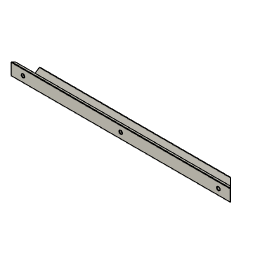
LightBar_Parametric (Autodesk Fusion 360 design; units mm, degrees)
Autodesk Fusion 360 part; units mm, degrees
note: some values were not read from the file. Set by a fixed rule: which sketch regions a step uses.
sketch "Sketch1" plane through (0, 0, 0) normal (1, 0, 0) x (0, 1, 0)
  line L0 (0, 0) -> (0, 15)
  line L1 (0, 0) -> (18, 0)
  line L2 (0, 15) -> (3, 15)
  line L3 (18, 0) -> (18, 9)
  line L4 (18, 9) -> (17.5385, 9)
  line L5 (17.5385, 9) -> (14.5385, 1.8)
  line L6 (14.5385, 1.8) -> (3, 6.6077)
  line L7 (3, 15) -> (3, 6.6077)
  dimension "d5" = 15
  dimension "d6" = 18
  dimension "d7" = 3
  dimension "d8" = 9
  dimension "d10" = 7.8
  dimension "d12" = 12.5
  dimension "d13" = 1.8
  constraint coincident L0.start L1.start
  constraint vertical L0
  constraint perpendicular L0 L1
  constraint perpendicular L0 L2
  constraint perpendicular L1 L3
  constraint perpendicular L3 L4
  constraint perpendicular L5 L6
  constraint vertical L7
  measures "d5" distance of L0.start L0.end
  measures "d6" distance of L0.start L1.end
  measures "d7" distance of L0.end L2.end
  measures "d8" distance of L1.end L3.end
  measures "d10" distance of L4.end L5.end
  measures "d12" distance of L5.end L6.end
  measures "d13" distance of L1 L5.end
extrude "Extrude1" add sketch "Sketch1" along normal blind 270
sketch "Sketch2" plane through (0, 0, 0) normal (0, 0, -1) x (1, 0, 0)
  line L0 (0, 0) -> (0, -18)
  line L1 (0, -18) -> (270, -18)
  line L2 (270, -18) -> (270, 0)
  line L3 (270, 0) -> (0, 0)
  line L4 (0, 0) -> (22.1271, 0) construction
  line L5 (0.05, 0) -> (18.05, -18)
  line L6 (269.95, 0) -> (251.95, -18)
  dimension "d35" = 45
  dimension "d36" = 0.05
  dimension "d37" = 0.05
  dimension "d38" = 45
  constraint horizontal L4
  constraint coincident L0.start L3.end
  constraint coincident L4 L5.start
  constraint coincident L1 L5.end
  constraint coincident L3 L6.start
  constraint coincident L1 L6.end
  measures "d35" angle of L4 L5
  measures "d36" distance of L0.start L5.start
  measures "d37" distance of L2.end L6.start
  measures "d38" angle of L3 L6
extrude "Extrude2" cut sketch "Sketch2" against normal through all contours L0 L1 L3 L5 | L1 L2 L3 L6
sketch "Sketch3" plane through (0, 0, 0) normal (0, -1, 0) x (1, 0, 0)
  line L0 (0.05, 0) -> (269.95, 0)
  line L1 (269.95, 15) -> (0.05, 15)
  line L2 (135, 0) -> (135, 15) construction
  circle A0 centre (135, 7.5) radius 1.8
  circle A1 centre (15, 7.5) radius 1.8
  circle A2 centre (255, 7.5) radius 1.8
  line L3 (269.95, 0) -> (269.95, 15)
  line L4 (0.05, 15) -> (0.05, 0)
  dimension "d19" = 3.6
  dimension "d22" = 120
  dimension "d23" = 0
  constraint midpoint L0 L2.start
  constraint midpoint L1 L2.end
  constraint midpoint L2 A0.centre
  measures "d19" diameter of A0
extrude "Extrude3" cut sketch "Sketch3" against normal blind 13 contours A0 | A1 | A2
sketch "Sketch4" plane through (0, 3, 0) normal (0, 1, 0) x (-1, 0, 0)
  arc A0 (-253.4367, 6.6077) -> (-256.5633, 6.6077) centre (-255, 7.5) ccw
  line L0 (-253.4367, 6.6077) -> (-136.5633, 6.6077)
  arc A1 (-133.4367, 6.6077) -> (-136.5633, 6.6077) centre (-135, 7.5) ccw
  line L1 (-133.4367, 6.6077) -> (-16.5633, 6.6077)
  arc A2 (-13.4367, 6.6077) -> (-16.5633, 6.6077) centre (-15, 7.5) ccw
  line L2 (-3.05, 15) -> (-266.95, 15)
  line L3 (-266.95, 6.6077) -> (-256.5633, 6.6077)
  circle A3 centre (-255, 7.5) radius 3.75
  circle A4 centre (-135, 7.5) radius 3.75
  circle A5 centre (-15, 7.5) radius 3.75
  line L4 (-13.4367, 6.6077) -> (-3.05, 6.6077)
  line L5 (-3.05, 6.6077) -> (-3.05, 15)
  line L6 (-266.95, 15) -> (-266.95, 6.6077)
  dimension "d26" = 7.5
  dimension "d27" = 7.5
  dimension "d28" = 7.5
  constraint concentric A0 A3
  constraint concentric A1 A4
  constraint concentric A2 A5
  measures "d26" diameter of A3
  measures "d27" diameter of A4
  measures "d28" diameter of A5
extrude "Extrude4" cut sketch "Sketch4" along normal blind 7 and the other way blind 1 contours A0 L0 L3 A3 | A0 L0 L3 A3 | L0 A1 L1 A4 | L0 A1 L1 A4 | L1 A2 A5 L4 | L1 A2 A5 L4
chamfer "Chamfer1" distance 0.4 angle 45 3 edges at (255, 3, 11.25) (135, 3, 11.25) (15, 3, 11.25) 3 faces at (4.44, 0, 7.5894) (91.0167, 1, 15) (96.0167, 6, 0)
equation "Angle1 = 45 °"
equation "Angle2 = 45 °"
equation "Clearance = 0.1 mm"
equation "Segment = 270 mm"
equation "d10 = d8 - 1.2 mm"
equation "d14 = Segment"
equation "d22 = ( Segment / 2 ) - 15 mm"
equation "d27 = d26"
equation "d28 = d26"
equation "d32 = 0.00 °"
equation "d35 = Angle2"
equation "d36 = Clearance / 2"
equation "d37 = Clearance / 2"
equation "d38 = Angle1"
